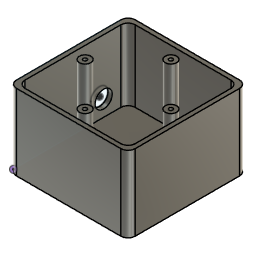
elektritarbijate_juhtimise_seade_korpus (Autodesk Fusion 360 design; units mm, degrees)
Autodesk Fusion 360 part; units mm, degrees
sketch "Sketch1" plane through (0, 0, 0) normal (0, 0, 1) x (1, 0, 0)
  line L0 (77, 0) -> (77, 77)
  line L1 (0, 77) -> (0, 0)
  line L2 (-3, 80) -> (80, 80)
  line L3 (80, 80) -> (80, -3)
  line L4 (80, -3) -> (-3, -3)
  line L5 (-3, -3) -> (-3, 80)
  line L6 (0, 0) -> (77, 0)
  line L7 (0, 77) -> (77, 77)
  line L8 (68.5, 8.5) -> (8.5, 8.5) construction
  line L9 (8.5, 8.5) -> (8.5, 68.5) construction
  line L10 (8.5, 68.5) -> (68.5, 68.5) construction
  line L11 (68.5, 68.5) -> (68.5, 8.5) construction
  circle A0 centre (38.5, 8.5) radius 1.35
  circle A1 centre (68.5, 38.5) radius 1.35
  circle A2 centre (8.5, 38.5) radius 1.35
  circle A3 centre (38.5, 68.5) radius 1.35
  circle A4 centre (38.5, 8.5) radius 4
  circle A5 centre (68.5, 38.5) radius 4
  circle A6 centre (38.5, 68.5) radius 4
  circle A7 centre (8.5, 38.5) radius 4
  line L12 (73, 18.8) -> (58, 18.8)
  line L13 (75, 0) -> (75, 20.8)
  line L14 (75, 20.8) -> (56, 20.8)
  line L15 (56, 20.8) -> (56, 0)
  line L16 (73, 18.8) -> (73, 3.3)
  line L17 (58, 18.8) -> (58, 3.3)
  line L18 (73, 3.3) -> (74, 3.3)
  line L19 (74, 3.3) -> (74, 0)
  line L20 (58, 3.3) -> (57, 3.3)
  line L21 (57, 3.3) -> (57, 0)
  line L22 (77, 46.5) -> (63.9, 46.5)
  line L23 (63.9, 46.5) -> (63.9, 71)
  line L24 (63.9, 71) -> (77, 71)
  line L25 (77, 71) -> (77, 46.5)
  line L26 (77, 44.5) -> (61.9, 44.5)
  line L27 (61.9, 44.5) -> (61.9, 73)
  line L28 (61.9, 73) -> (77, 73)
  line L29 (4, 0) -> (33.7, 0)
  line L30 (33.7, 0) -> (33.7, 4.2)
  line L31 (33.7, 4.2) -> (4, 4.2)
  line L32 (4, 4.2) -> (4, 0)
  line L33 (6, 4.2) -> (6, 2.35)
  line L34 (6, 2.35) -> (31.6, 2.35)
  line L35 (4, 4.2) -> (4, 6.2)
  line L36 (31.6, 2.35) -> (31.6, 4.2)
  line L37 (4, 6.2) -> (33.7, 6.2)
  line L38 (33.7, 6.2) -> (33.7, 4.2)
  dimension "d1" = 77
  dimension "d2" = 77
  dimension "d36" = 3
  dimension "d39" = 3
  dimension "d104" = 3
  dimension "d105" = 3
  dimension "d110" = 60
  dimension "d111" = 60
  dimension "d114" = 8.5
  dimension "d115" = 8.5
  dimension "d116" = 2.7
  dimension "d117" = 2.7
  dimension "d118" = 2.7
  dimension "d119" = 2.7
  dimension "d120" = 8
  dimension "d121" = 8
  dimension "d122" = 8
  dimension "d123" = 8
  dimension "d140" = 15
  dimension "d142" = 20.8
  dimension "d145" = 15.5
  dimension "d146" = 15.5
  dimension "d147" = 1
  dimension "d148" = 1
  dimension "d149" = 2
  dimension "d150" = 2
  dimension "d151" = 2
  dimension "d152" = 2
  dimension "d164" = 13.1
  dimension "d165" = 24.5
  dimension "d166" = 2
  dimension "d167" = 2
  dimension "d168" = 2
  dimension "d169" = 4
  dimension "d174" = 29.7
  dimension "d175" = 4.2
  dimension "d176" = 4
  dimension "d177" = 1.85
  dimension "d179" = 2
  dimension "d180" = 2
  dimension "d182" = 2.1
  dimension "d185" = 29.7
  constraint vertical L0
  constraint vertical L1
  constraint coincident L1.end L6.start
  constraint horizontal L2
  constraint vertical L3
  constraint horizontal L4
  constraint vertical L5
  constraint perpendicular L0 L6
  constraint perpendicular L0 L7
  constraint horizontal L8
  constraint vertical L9
  constraint horizontal L10
  constraint vertical L11
  constraint midpoint L8 A0.centre
  constraint midpoint L11 A1.centre
  constraint midpoint L9 A2.centre
  constraint midpoint L10 A3.centre
  constraint concentric A0 A4
  constraint concentric A1 A5
  constraint concentric A3 A6
  constraint concentric A2 A7
  constraint coincident L6 L13.start
  constraint perpendicular L6 L13
  constraint perpendicular L13 L14
  constraint coincident L6 L15.end
  constraint perpendicular L6 L15
  constraint perpendicular L12 L16
  constraint perpendicular L12 L17
  constraint perpendicular L0 L18
  constraint coincident L6 L19.end
  constraint perpendicular L6 L19
  constraint perpendicular L17 L20
  constraint coincident L6 L21.end
  constraint perpendicular L6 L21
  constraint horizontal L22
  constraint vertical L23
  constraint horizontal L24
  constraint vertical L25
  constraint coincident L0 L22.start
  constraint coincident L0 L26.start
  constraint perpendicular L0 L26
  constraint perpendicular L22 L27
  constraint coincident L0 L28.end
  constraint perpendicular L27 L28
  constraint horizontal L29
  constraint vertical L30
  constraint horizontal L31
  constraint vertical L32
  constraint coincident L6 L29.start
  constraint coincident L31 L33.start
  constraint perpendicular L31 L33
  constraint perpendicular L33 L34
  constraint perpendicular L31 L35
  constraint coincident L31 L36.end
  constraint perpendicular L31 L36
  constraint perpendicular L35 L37
  measures "d1" distance of L1.end L0.start
  measures "d2" distance of L1.end L1.start
  measures "d36" distance of L0 L3
  measures "d39" distance of L1 L5
  measures "d104" distance of L2 L7
  measures "d105" distance of L4 L6
  measures "d110" distance of L8.start L8.end
  measures "d111" distance of L8.start L10.end
  measures "d114" distance of L0 L11
  measures "d115" distance of L6 L8
  measures "d116" diameter of A0
  measures "d117" diameter of A1
  measures "d118" diameter of A2
  measures "d119" diameter of A3
  measures "d120" diameter of A4
  measures "d121" diameter of A5
  measures "d122" diameter of A6
  measures "d123" diameter of A7
  measures "d140" distance of L12.start L12.end
  measures "d142" distance of L13.start L13.end
  measures "d145" distance of L12.start L16.end
  measures "d146" distance of L12.end L17.end
  measures "d147" distance of L16.end L18.end
  measures "d148" distance of L17.end L20.end
  measures "d149" distance of L15 L17
  measures "d150" distance of L13 L16
  measures "d151" distance of L0 L13
  measures "d152" distance of L12 L14
  measures "d164" distance of L22.start L22.end
  measures "d165" distance of L22.start L24.end
  measures "d166" distance of L24 L28
  measures "d167" distance of L23 L27
  measures "d168" distance of L22 L26
  measures "d169" distance of L7 L28
  measures "d174" distance of L29.start L29.end
  measures "d175" distance of L29.start L31.end
  measures "d176" distance of L1 L32
  measures "d177" distance of L33.start L33.end
  measures "d179" distance of L32 L33
  measures "d180" distance of L31.end L35.end
  measures "d182" distance of L30 L36
  measures "d185" distance of L35.end L37.end
extrude "Extrude1" add sketch "Sketch1" along normal blind 3 contours L0 L1 L6 L7 L13 L14 L15 L26 L27 L28 L30 L32 L35 L37 L38 | L0 L22 L23 L24 L26 L27 L28 | L6 L12 L13 L14 L15 L16 L17 L18 L19 L20 L21 | L0 L22 L23 L24 L25 | L6 L12 L16 L17 L18 L19 L20 L21 | L6 L29 L30 L31 L32 L33 L34 L36 | L31 L35 L37 L38 | L31 L33 L34 L36 | L2 L3 L4 L5 | A0 | A1 | A2 | A3 | A4 | A5 | A6 | A7 makes body 1
extrude "Extrude2" add sketch "Sketch1" along normal blind 53 contours L2 L3 L4 L5 bodies 1
fillet "Fillet7" radius 5 4 edges at (-3, -3, 26.5) (80, -3, 26.5) (-3, 80, 26.5) (80, 80, 26.5) on bodies 1
fillet "Fillet8" radius 5 4 edges at (0, 77, 28) (0, 0, 28) (77, 0, 28) (77, 77, 28) on bodies 1
extrude "Extrude6" add sketch "Sketch1" along normal blind 50 from surface at 3 contours A4 | A5 | A6 | A7 bodies 1
extrude "Extrude7" add sketch "Sketch1" along normal blind 33 separate body contours A0 | A1 | A2 | A3 makes body 2 at (39.8433, 8.3656, 22) makes body 3 at (7.1517, 38.4327, 22) makes body 4 at (68.4663, 39.8496, 22) makes body 5 at (39.8083, 68.8331, 22)
chamfer "Chamfer2" distance 2 angle 45 4 edges at (34.7707, 69.9465, 3) (64.7707, 39.9465, 3) (34.7707, 9.9465, 3) (4.7707, 39.9465, 3) on bodies 1
sketch "Sketch3" plane through (-3, 0, 0) normal (-1, 0, 0) x (0, -1, 0)
  line L0 (-75, 53) -> (-75, 0)
  line L1 (-75, 0) -> (-2, 0)
  line L2 (-2, 0) -> (-2, 53)
  line L3 (-2, 53) -> (-75, 53)
  circle A0 centre (-60, 14) radius 6
  dimension "d134" = 12
  dimension "d135" = 60
  dimension "d136" = 14
  measures "d134" diameter of A0
  measures "d135" horizontal distance of origin A0.centre
  measures "d136" vertical distance of origin A0.centre
extrude "Extrude8" cut sketch "Sketch3" against normal blind 4 contours A0 bodies 1
extrude "Extrude9" add sketch "Sketch1" along normal blind 33 separate body contours L6 L12 L13 L14 L15 L16 L17 L18 L19 L20 L21 makes body 6
sketch "Sketch4" plane through (0, 18.8, 0) normal (0, -1, 0) x (1, 0, 0)
  line L0 (58, 0) -> (73, 0)
  line L1 (73, 0) -> (73, 33)
  line L2 (73, 33) -> (58, 33)
  line L3 (58, 33) -> (58, 0)
  line L4 (60, 3) -> (70, 3)
  line L5 (70, 3) -> (70, 10.5)
  line L6 (60, 10.5) -> (60, 3)
  arc A0 (65, 15.5) -> (60, 10.5) centre (65, 10.5) ccw
  arc A1 (70, 10.5) -> (65, 15.5) centre (65, 10.5) ccw
  dimension "d155" = 2
  dimension "d156" = 3
  dimension "d157" = 10
  dimension "d159" = 5
  constraint horizontal L4
  constraint vertical L5
  constraint vertical L6
  constraint tangent L6 A0
  constraint tangent L5 A1
  constraint equal A0 A1
  constraint coincident A0.start A1.end
  measures "d155" distance of L3 L6
  measures "d156" distance of L0 L4
  measures "d157" distance of L5 L6
  measures "d159" radius of A0
extrude "Extrude10" cut sketch "Sketch4" against normal blind 2 contours L4 L5 L6 A0 A1 bodies 6
fillet "Fillet9" radius 2 2 edges at (56, 20.8, 16.5) (75, 20.8, 16.5) on bodies 6
extrude "Extrude11" add sketch "Sketch1" along normal blind 17 separate body contours L0 L22 L23 L24 L26 L27 L28 makes body 7
fillet "Fillet10" radius 2 2 edges at (61.9, 44.5, 8.5) (61.9, 73, 8.5) on bodies 7
extrude "Extrude12" add sketch "Sketch1" along normal blind 10 separate body contours L6 L29 L30 L31 L32 L33 L34 L36 | L31 L35 L37 L38 makes body 8
combine "Combine1" operation add target body 4 tool bodies 1 8 6 2 7 5 3
equation "d145 = 18.8 mm - 3.3 mm"
equation "d146 = 18.8 mm - 3.3 mm"
